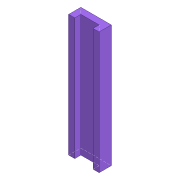
# Autodesk Inventor part: Bancada
Saved by Autodesk Inventor 2021 (Build 250183000, 183)
## iProperties
Created: 2021-10-18
Part Number: Bancada
Material: Steel
Document SubType Name: Modeling
Designer: Usuario
Density: 7.85 g/cm^3
Appearance: Violet
Author: Usuario
Autodesk Inventor part; units mm, degrees
ref_plane "YZ Plane" through (0, 0, 0) normal (1, 0, 0) x (0, 1, 0)
ref_plane "XZ Plane" through (0, 0, 0) normal (0, 1, 0) x (-1, 0, 0)
ref_plane "XY Plane" through (0, 0, 0) normal (0, 0, 1) x (1, 0, 0)
sketch "Sketch1" plane through (0, 0, 0) normal (0, 1, 0) x (-1, 0, 0)
  line L0 (15, 5) -> (-15, 5) construction
  line L1 (-15, 5) -> (-15, -5)
  line L2 (-15, -5) -> (15, -5)
  line L3 (15, -5) -> (15, 5)
  line L4 (15, 5) -> (-15, -5) construction
  line L5 (-15, 5) -> (15, -5) construction
  line L6 (15, 5) -> (25, 5)
  line L7 (25, 5) -> (25, -15)
  line L8 (25, -15) -> (-25, -15)
  line L9 (-25, -15) -> (-25, 5)
  line L10 (-25, 5) -> (-15, 5)
  point P0 (0, 0)
  dimension "d0" = 30
  dimension "d1" = 10
  dimension "d2" = 10
  dimension "d3" = 10
  dimension "d4" = 10
  constraints: 22 end point, 5 perpendicular, 2 horizontal, 2 midpoint, 2 parallel, 1 point on line
  measures "d0" distance of L2.end L1.end
  measures "d1" distance of L1.end L0.end
  measures "d2" distance of L0.start L6.end
  measures "d3" distance of L9.end L0.end
  measures "d4" distance between parallel lines of L2 L8
extrude "Extrusion1" add sketch "Sketch1" along normal mid plane 200
body "Solid1"
